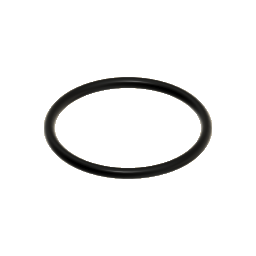
Rubber_22mm (Autodesk Fusion 360 design; units mm, degrees)
Autodesk Fusion 360 part; units mm, degrees
sketch "Sketch1" plane through (0, 0, 0) normal (0, 0, 1) x (1, 0, 0)
  circle A0 centre (0, 0) radius 11
  circle A1 centre (0, 0) radius 9.5
  dimension "d1" = 22
  dimension "d2" = 19
  constraint coincident A0.centre A1.centre
  measures "d1" diameter of A0
  measures "d2" diameter of A1
extrude "Extrude1" add sketch "Sketch1" along normal blind 1.5
fillet "Fillet1" radius 0.75 4 edges at (-10.2556, -3.9778, 1.5) (-10.2556, -3.9778, 0) (-8.8571, 3.4353, 1.5) (-8.8571, 3.4353, 0)
equation "d1 = outerDiameter"
equation "d2 = innerDiameter"
equation "d3 = height"
equation "d6 = height / 2"
equation "outerDiameter = 22 mm"
equation "innerDiameter = 19 mm"
equation "height = 1.5 mm"
named bodies: "Rubber_10mm"
